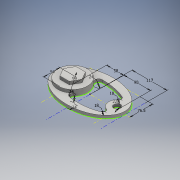
# Autodesk Inventor part: 스케치03
Saved by Autodesk Inventor 2016 (Build 200138000, 138)
## iProperties
Created: 2024-04-19
Part Number: 스케치03
Material: 일반
Document SubType Name: Modeling
Designer: pc
Density: 1 g/cm^3
Appearance: 기본값
Author: pc
Autodesk Inventor part; units mm, degrees
ref_plane "YZ Plane" through (0, 0, 0) normal (1, 0, 0) x (0, 1, 0)
ref_plane "XZ Plane" through (0, 0, 0) normal (0, 1, 0) x (-1, 0, 0)
ref_plane "XY Plane" through (0, 0, 0) normal (0, 0, 1) x (1, 0, 0)
sketch "스케치1" plane through (0, 0, 0) normal (0, 0, 1) x (1, 0, 0)
  point P0 (0, 0)
sketch "스케치2" plane through (0, 0, 0) normal (0, 0, 1) x (1, 0, 0)
  line L0 (-99.4603, 0.601) -> (134.5397, 0.601) construction
  circle A0 centre (-57.9969, 0.601) radius 49.5
  circle A1 centre (90, 0.601) radius 11
  line L1 (-73.5853, 27.601) -> (-42.4084, 27.601)
  line L2 (-42.4084, 27.601) -> (-26.82, 0.601)
  line L3 (-26.82, 0.601) -> (-42.4084, -26.399)
  line L4 (-42.4084, -26.399) -> (-73.5853, -26.399)
  line L5 (-73.5853, -26.399) -> (-89.1738, 0.601)
  line L6 (-89.1738, 0.601) -> (-73.5853, 27.601)
  line L7 (-58.042, 84.9456) -> (-58.042, -105.8358) construction
  line L8 (89.9996, 81.1974) -> (89.9996, -76.9686) construction
  arc A2 (-20.975, -32.2567) -> (-13.3377, -52.1475) centre (-12, -40.2222) ccw
  arc A3 (79.0529, -41.2883) -> (78.3038, -24.1379) centre (75.9743, -32.8313) ccw
  arc A4 (72.8199, 21.9003) -> (71.1275, 36.8763) centre (67.084, 28.8357) ccw
  ellipse E0 centre (0, 0) end of major axis (-117, -0.0052) minor radius 77.101
  line L9 (117, 66.3742) -> (117, -80.3168) construction
  line L10 (-78.2443, 77.101) -> (89.9996, 77.101) construction
  line L11 (0, 100.1745) -> (0, -148.4389) construction
  arc A5 (-12.0086, 53.4242) -> (-20.975, 33.4587) centre (-12, 41.4242) ccw
  ellipse E1 centre (0, 0) end of major axis (-110.153, 7.6024) minor radius 53.1482 (-13.3377, -52.1475) -> (80.2954, -40.7261) ccw
  ellipse E2 centre (0, 0) end of major axis (-110.1827, 7.465) minor radius 53.0214 (71.1275, 36.8763) -> (-12.0086, 53.4242) ccw
  arc A6 (116.9989, 0.3429) -> (117, 0.6731) centre (90, 0.601) ccw
  arc A7 (72.8199, 21.9003) -> (80.5446, -25.078) centre (90, 0.601) ccw
  point P0 (0, 52.7518)
  point P1 (0, 52.7518)
  point P2 (0, 52.7518)
  point P3 (0, 52.7518)
  point P4 (0, 52.7518)
  point P5 (0, 52.7518)
  point P6 (0, 52.7518)
  point P7 (0, 52.7518)
  point P8 (0, 52.7518)
  point P9 (0, 52.7518)
  point P10 (0, 52.7518)
  point P11 (0, 52.7518)
  point P12 (0, 77.101)
  point P13 (0, 52.7518)
  point P14 (0, -77.101)
  point P15 (0, -52.7518)
  point P16 (0, -52.7518)
  point P17 (0, -77.101)
  point P18 (0, -52.7518)
  point P19 (0, -52.7518)
  point P20 (0, -52.7518)
  point P21 (32.4105, -49.2482)
  point P22 (0, -52.7518)
  point P23 (0, -52.7518)
  point P24 (0, -53.101)
  point P25 (0, -77.101)
  dimension "d3" = 99
  dimension "d4" = 58
  dimension "d5" = 22
  dimension "d6" = 54
  dimension "d7" = 90
  dimension "d9" = 24
  dimension "d11" = 18
  dimension "d12" = 18
  dimension "d14" = 76.5
  dimension "d16" = 117
  dimension "d18" = 24
  dimension "d21" = 24
  constraints: 22 end point, 21 coincident, 18 point on circle, 8 centre point, 5 point on line, 4 vertical, 3 horizontal, 2 tangent, 1 perpendicular, 39 other
  measures "d3" diameter of A0
  measures "d4" distance of point (0, 0) A0.centre
  measures "d5" diameter of A1
  measures "d6" distance between parallel lines of L4 L1
  measures "d7" horizontal distance of A1.centre point (0, 0)
  measures "d9" diameter of A2
  measures "d11" diameter of A3
  measures "d12" diameter of A4
  measures "d14" distance between parallel lines of L0 L10
  measures "d16" distance of the line from the sketch origin of L9
  measures "d18" diameter of A5
  measures "d21" distance of point (0, -53.101) point (0, -77.101)
extrude "돌출1" add sketch "스케치2" along normal blind 10 contours E0
extrude "돌출2" add sketch "스케치2" along normal blind 20 contours A0
extrude "돌출3" add sketch "스케치2" along normal blind 30 contours L1 L2 L3 L4 L5 L6
